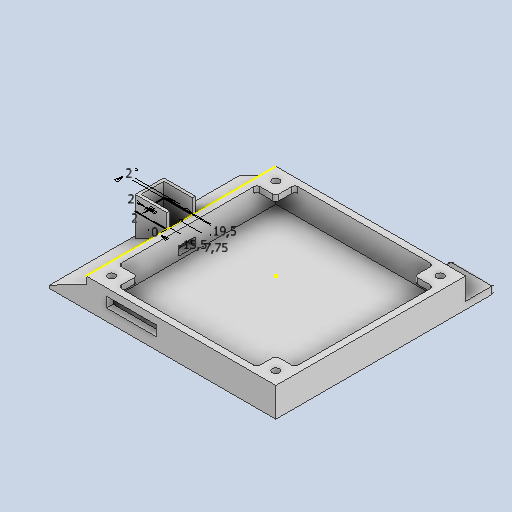
# Autodesk Inventor part: bottom
Saved by Autodesk Inventor 2025 (Build 290162000, 162)
## iProperties
Created: 2025-08-22
Part Number: bottom
Material: Generic
Document SubType Name: Modeling
Designer: Pravoslav
Density: 1 g/cm^3
Appearance: Default
Author: Pravoslav
Autodesk Inventor part; units mm, degrees
ref_plane "YZ Plane" through (0, 0, 0) normal (1, 0, 0) x (0, 1, 0)
ref_plane "XZ Plane" through (0, 0, 0) normal (0, 1, 0) x (-1, 0, 0)
ref_plane "XY Plane" through (0, 0, 0) normal (0, 0, 1) x (1, 0, 0)
sketch "Sketch1" plane through (0, 0, 0) normal (0, 1, 0) x (-1, 0, 0)
  line L0 (65, 65) -> (-65, 65)
  line L1 (-65, 65) -> (-65, -65)
  line L2 (-65, -65) -> (65, -65)
  line L3 (65, -65) -> (65, 65)
  line L4 (65, 65) -> (-65, -65) construction
  line L5 (-65, 65) -> (65, -65) construction
  line L6 (65, 65) -> (90, 65)
  line L7 (90, 65) -> (90, -65)
  line L8 (90, -65) -> (65, -65)
  line L9 (65, -65) -> (65, 65)
  point P0 (0, 0)
  dimension "d0" = 130
  dimension "d1" = 130
  dimension "d2" = 25
  dimension "d3" = 130
  constraints: 20 end point, 4 parallel, 2 horizontal, 2 midpoint, 2 perpendicular
  measures "d0" distance of L2.end L1.end
  measures "d1" distance of L1.end L0.end
  measures "d2" distance of L7.end L8.end
  measures "d3" distance between parallel lines of L8 L6
extrude "Extrusion1" add sketch "Sketch1" along normal blind 2
sketch "Sketch2" plane through (0, 2, 0) normal (0, 1, 0) x (1, 0, 0)
  line L0 (-65, -65) -> (65, -65)
  line L1 (65, -65) -> (65, 65)
  line L2 (65, 65) -> (-65, 65)
  line L3 (-65, 65) -> (-65, -65)
  line L4 (-65, -65) -> (65, 65) construction
  line L5 (65, -65) -> (-65, 65) construction
  line L6 (-60.5, -60.5) -> (60.5, -60.5)
  line L7 (60.5, -60.5) -> (60.5, 60.5)
  line L8 (60.5, 60.5) -> (-60.5, 60.5)
  line L9 (-60.5, 60.5) -> (-60.5, -60.5)
  line L10 (-60.5, -60.5) -> (60.5, 60.5) construction
  line L11 (60.5, -60.5) -> (-60.5, 60.5) construction
  point P0 (0, 0)
  dimension "d6" = 130
  dimension "d7" = 130
  dimension "d8" = 4.5
  dimension "d9" = 4.5
  constraints: 24 end point, 4 midpoint, 4 parallel, 2 horizontal, 2 perpendicular
  measures "d6" distance of L2.end L1.end
  measures "d7" distance of L1.end L0.end
  measures "d8" distance between parallel lines of L2 L8
  measures "d9" distance between parallel lines of L1 L7
extrude "Extrusion2" add sketch "Sketch2" along normal blind 18
sketch "Sketch3" plane through (0, 20, 0) normal (0, 1, 0) x (1, 0, 0)
  line L0 (65, -65) -> (65, 65) projected
  line L1 (65, -65) -> (47.5, -65)
  line L2 (47.5, -65) -> (47.5, -47.5)
  line L3 (47.5, -47.5) -> (65, -47.5)
  line L4 (65, -47.5) -> (65, -65)
  line L5 (-65, -65) -> (-47.5, -65)
  line L6 (-47.5, -65) -> (-47.5, -47.5)
  line L7 (-47.5, -47.5) -> (-65, -47.5)
  line L8 (-65, -47.5) -> (-65, -65)
  line L9 (-65, 65) -> (-47.5, 65)
  line L10 (-47.5, 65) -> (-47.5, 47.5)
  line L11 (-47.5, 47.5) -> (-65, 47.5)
  line L12 (-65, 47.5) -> (-65, 65)
  line L13 (65, 65) -> (47.5, 65)
  line L14 (47.5, 65) -> (47.5, 47.5)
  line L15 (47.5, 47.5) -> (65, 47.5)
  line L16 (65, 47.5) -> (65, 65)
  circle A0 centre (56.25, -56.25) radius 2.5
  circle A1 centre (56.25, 56.25) radius 2.5
  circle A2 centre (-56.25, 56.25) radius 2.5
  circle A3 centre (-56.25, -56.25) radius 2.5
  line L17 (-65, 65) -> (-65, -65) projected
  point P0 (0, 0)
  point P1 (-47.5, 56.25)
  point P2 (47.5, -56.25)
  point P3 (56.25, -47.5)
  dimension "d12" = 17.5
  dimension "d13" = 17.5
  dimension "d14" = 17.5
  dimension "d15" = 17.5
  dimension "d16" = 17.5
  dimension "d17" = 17.5
  dimension "d18" = 17.5
  dimension "d19" = 17.5
  dimension "d20" = 5
  dimension "d21" = 5
  dimension "d22" = 5
  dimension "d23" = 5
  dimension "d24" = 8.75
  dimension "d25" = 8.75
  dimension "d26" = 17.5
  dimension "d27" = 8.75
  dimension "d28" = 8.75
  dimension "d29" = 8.75
  dimension "d30" = 8.75
  dimension "d31" = 8.75
  dimension "d32" = 8.75
  constraints: 32 end point, 8 parallel, 4 centre point, 4 horizontal, 4 perpendicular, 3 midpoint, 2 point on line
  measures "d12" distance of L2.end L3.end
  measures "d13" distance of L7.end L6.end
  measures "d14" distance of L6.end L5.end
  measures "d15" distance of L10.end L11.end
  measures "d16" distance of L9.end L10.end
  measures "d17" distance of L15.end L14.end
  measures "d18" distance of L14.end L13.end
  measures "d19" distance between parallel lines of L1 L3
  measures "d20" diameter of A0
  measures "d21" diameter of A1
  measures "d22" diameter of A2
  measures "d23" diameter of A3
  measures "d24" distance from line of L6 A3.centre
  measures "d25" distance from line of L7 A3.centre
  measures "d26" distance between parallel lines of L17 L6
  measures "d27" distance of point (-47.5, 56.25) A2.centre
  measures "d28" distance from line of L11 A2.centre
  measures "d29" distance from line of L14 A1.centre
  measures "d30" distance from line of L15 A1.centre
  measures "d31" distance of point (47.5, -56.25) A0.centre
  measures "d32" distance of point (56.25, -47.5) A0.centre
extrude "Extrusion3" add sketch "Sketch3" against normal blind 4
fillet "Fillet1" radius 2 3 edges at (47.5, 18, 60.5) (60.5, 18, 47.5) (47.5, 18, 47.5)
mirror "Mirror1" about plane through (0, 0, 0) normal (1, 0, 0) of "Fillet1"
mirror "Mirror2" about plane through (0, 0, 0) normal (0, 0, 1) of "Fillet1", "Mirror1"
chamfer "Chamfer1" distance 25 distance2 13 1 edges at (-65, 2, 0) measured on face at (-65.5, 2, 0)
sketch "Sketch5" plane through (-90, 0, 65) normal (0, 0, 1) x (1, 0, 0)
  line L0 (39, 15) -> (73, 15)
  line L1 (73, 15) -> (73, 8)
  line L2 (73, 8) -> (39, 8)
  line L3 (39, 8) -> (39, 15)
  line L4 (25, 20) -> (155, 20) projected
  line L5 (25, 2) -> (25, 20) projected
  point P0 (90, 0)
  dimension "d42" = 34
  dimension "d43" = 7
  dimension "d44" = 5
  dimension "d45" = 14
  constraints: 8 end point, 2 parallel, 1 horizontal, 1 perpendicular
  measures "d42" distance between parallel lines of L1 L3
  measures "d43" distance between parallel lines of L2 L0
  measures "d44" distance between parallel lines of L4 L0
  measures "d45" distance between parallel lines of L5 L3
extrude "Extrusion5" cut sketch "Sketch5" against normal blind 10
sketch "Sketch9" plane through (0, 0, 0) normal (0, -1, 0) x (1, 0, 0)
  line L0 (65, 65) -> (65, -65) projected
  line L1 (65, -65) -> (35, -65)
  line L2 (35, -65) -> (35, -85)
  line L3 (35, -85) -> (65, -85)
  line L4 (65, -85) -> (65, -65)
  circle A0 centre (50, -75) radius 2.75
  point P0 (0, 0)
  dimension "d66" = 30
  dimension "d67" = 20
  dimension "d68" = 5.5
  constraints: 8 end point, 2 parallel, 1 centre point, 1 horizontal, 1 perpendicular
  measures "d66" distance of L3.end L2.end
  measures "d67" distance of L2.end L1.end
  measures "d68" diameter of A0
extrude "Extrusion9" add sketch "Sketch9" against normal blind 5
fillet "Fillet3" radius 2 5 edges at (65, 2.5, -85) (35, 2.5, -85) (50, 5, -85) (35, 5, -75) (35, 2.5, -65)
sketch "Sketch10" plane through (0, 20, 0) normal (0, 1, 0) x (1, 0, 0)
  line L0 (-65, 65) -> (-65, -65) projected
  line L1 (-65, 7.75) -> (-84.5, 7.75)
  line L2 (-84.5, 7.75) -> (-84.5, -7.75)
  line L3 (-84.5, -7.75) -> (-65, -7.75)
  line L4 (-65, -7.75) -> (-65, 7.75)
  line L5 (-65, 9.75) -> (-86.5, 9.75)
  line L6 (-86.5, 9.75) -> (-86.5, -9.75)
  line L7 (-86.5, -9.75) -> (-65, -9.75)
  line L8 (-65, -9.75) -> (-65, 9.75)
  point P0 (0, 0)
  point P1 (-65, 0)
  point P2 (-75.75, 9.75)
  dimension "d72" = 19.5
  dimension "d73" = 15.5
  dimension "d74" = 7.75
  dimension "d75" = 2
  dimension "d76" = 2
  dimension "d77" = 0
  dimension "d78" = 2
  constraints: 16 end point, 4 parallel, 2 horizontal, 2 midpoint, 2 perpendicular, 1 point on line
  measures "d72" distance between parallel lines of L0 L2
  measures "d73" distance between parallel lines of L3 L1
  measures "d74" distance from line of point (-65, 0) L1
  measures "d75" distance from line of L1 point (-75.75, 9.75)
  measures "d76" distance between parallel lines of L6 L2
  measures "d77" distance between parallel lines of L0 L8
  measures "d78" distance between parallel lines of L3 L7
extrude "Extrusion10" add sketch "Sketch10" along normal up to surface contours L0 L1 L2 L3 L7 L6 L5 surface through (-77.5, 8.5, -32.5) normal (-0.4613527, 0.8872168, 0)
extrude "Extrusion11" cut sketch "Sketch10" against normal up to surface (18 mm away) contours L0 L3 L2 L1
extrude "Extrusion12" add sketch "Sketch10" along normal blind 10 contours L0 L1 L2 L3 L7 L6 L5
sketch "Sketch11" plane through (-60.5, 2, 60.5) normal (1, 0, 0) x (0, 0, -1)
  line L0 (54.6068, 8.4352) -> (65.6416, 8.4352)
  line L1 (65.6416, 8.4352) -> (65.6416, 2.4891)
  line L2 (65.6416, 2.4891) -> (54.6068, 2.4891)
  line L3 (54.6068, 2.4891) -> (54.6068, 8.4352)
  point P0 (60.5, -2)
  constraints: 8 end point, 2 parallel, 1 horizontal, 1 perpendicular
extrude "Extrusion13" cut sketch "Sketch11" against normal blind 10
sketch "Sketch4" plane through (65, 0, -65) normal (0, 0, -1) x (-1, 0, 0)
  line L0 (82, 10) -> (116, 10)
  line L1 (116, 10) -> (116, 3)
  line L2 (116, 3) -> (82, 3)
  line L3 (82, 3) -> (82, 10)
  line L4 (0, 20) -> (130, 20) projected
  line L5 (130, 2) -> (130, 20) projected
  point P0 (65, 0)
  dimension "d36" = 7
  dimension "d37" = 34
  dimension "d38" = 5
  dimension "d39" = 14
  constraints: 8 end point, 2 parallel, 1 horizontal, 1 perpendicular
  measures "d36" distance between parallel lines of L2 L0
  measures "d37" distance between parallel lines of L1 L3
  measures "d39" distance between parallel lines of L5 L1
sketch "Sketch8" plane through (0, 0, 0) normal (0, -1, 0) x (1, 0, 0)
  line L0 (65, 65) -> (35, 65)
  line L1 (35, 65) -> (35, 85)
  line L2 (35, 85) -> (65, 85)
  line L3 (65, 85) -> (65, 65)
  circle A0 centre (50, 75) radius 2.75
  point P0 (0, 0)
  dimension "d58" = 30
  dimension "d59" = 20
  dimension "d60" = 5.5
  dimension "d61" = 15
  dimension "d62" = 10
  constraints: 8 end point, 2 parallel, 1 centre point, 1 horizontal, 1 perpendicular
  measures "d58" distance of L1.end L2.end
  measures "d59" distance of L0.end L1.end
  measures "d60" diameter of A0
  measures "d61" distance from line of L3 A0.centre
  measures "d62" distance from line of L0 A0.centre
sketch "Sketch6" plane through (0, 0, 0) normal (0, -1, 0) x (1, 0, 0)
  line L0 (-65, -65) -> (-65, 65) projected
  circle A0 centre (-77.5, 0) radius 3
  line L1 (-90, -65) -> (-90, 65) projected
  point P0 (0, 0)
  dimension "d51" = 6
  dimension "d52" = 12.5
  constraints: 1 centre point
  measures "d51" diameter of A0
  measures "d52" distance from line of L1 A0.centre
sketch "Sketch7" plane through (0, 20, 0) normal (0, 1, 0) x (1, 0, 0)
  circle A0 centre (-77.5, 0) radius 3 projected
  circle A1 centre (-77.5, 0) radius 6
  point P0 (0, 0)
  dimension "d55" = 12
  constraints: 1 centre point, 1 coincident
  measures "d55" diameter of A1
body "Solid1"
